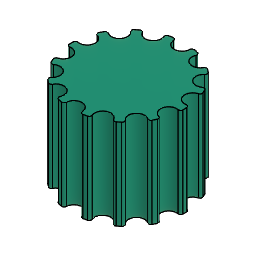
14T Pulley template v3 (Autodesk Fusion 360 design; units mm, degrees)
Autodesk Fusion 360 part; units mm, degrees
sketch "Sketch1" plane through (0, 0, 0) normal (0, 0, 1) x (1, 0, 0)
  circle A0 centre (0, 0) radius 6.305 construction
  circle A1 centre (0, 0) radius 5.105 construction
  line L0 (0, 0) -> (0, 5.105) construction
  circle A2 centre (0, 5.995) radius 0.89 construction
  circle A3 centre (1.139, 5.9469) radius 0.25 construction
  line L1 (0, 0) -> (2.7356, 5.6806) construction
  line L2 (0, 0) -> (6.305, 0) construction
  circle A4 centre (2.6011, 5.4013) radius 0.89 construction
  circle A5 centre (1.5541, 5.8522) radius 0.25 construction
  arc A6 (0.9079, 5.9375) -> (0.8892, 5.9575) centre (0, 5.105) ccw construction
  arc A7 (0, 5.105) -> (0.8892, 5.9575) centre (0, 5.995) ccw
  arc A8 (1.186, 6.1924) -> (0.8892, 5.9575) centre (1.139, 5.9469) ccw
  arc A9 (1.7837, 5.7533) -> (1.6182, 6.0938) centre (1.5541, 5.8522) ccw
  arc A10 (1.7837, 5.7533) -> (2.215, 4.5994) centre (2.6011, 5.4013) ccw
  line L3 (1.186, 6.1924) -> (1.6182, 6.0938)
  arc A11 (-0.8892, 5.9575) -> (0, 5.105) centre (0, 5.995) ccw
  arc A12 (-0.8892, 5.9575) -> (-1.186, 6.1924) centre (-1.139, 5.9469) ccw
  line L4 (-1.6182, 6.0938) -> (-1.186, 6.1924)
  arc A13 (-1.6182, 6.0938) -> (-1.7837, 5.7533) centre (-1.5541, 5.8522) ccw
  arc A14 (-2.215, 4.5994) -> (-1.7837, 5.7533) centre (-2.6011, 5.4013) ccw
  arc A15 (-3.386, 4.9817) -> (-2.215, 4.5994) centre (-2.6011, 5.4013) ccw
  arc A16 (-3.386, 4.9817) -> (-3.7554, 5.0646) centre (-3.6065, 4.8638) ccw
  line L5 (-4.102, 4.7882) -> (-3.7554, 5.0646)
  arc A17 (-4.102, 4.7882) -> (-4.1033, 4.4096) centre (-3.9393, 4.5983) ccw
  arc A18 (-3.9912, 3.1829) -> (-4.1033, 4.4096) centre (-4.6871, 3.7378) ccw
  arc A19 (-5.2121, 3.0192) -> (-3.9912, 3.1829) centre (-4.6871, 3.7378) ccw
  arc A20 (-5.2121, 3.0192) -> (-5.5809, 2.9337) centre (-5.3596, 2.8173) ccw
  line L6 (-5.7733, 2.5342) -> (-5.5809, 2.9337)
  arc A21 (-5.7733, 2.5342) -> (-5.6102, 2.1926) centre (-5.5444, 2.4337) ccw
  arc A22 (-4.977, 1.136) -> (-5.6102, 2.1926) centre (-5.8447, 1.334) ccw
  arc A23 (-6.006, 0.4587) -> (-4.977, 1.136) centre (-5.8447, 1.334) ccw
  arc A24 (-6.006, 0.4587) -> (-6.3011, 0.2217) centre (-6.0513, 0.2129) ccw
  line L7 (-6.3011, -0.2217) -> (-6.3011, 0.2217)
  arc A25 (-6.3011, -0.2217) -> (-6.006, -0.4587) centre (-6.0513, -0.2129) ccw
  arc A26 (-4.977, -1.136) -> (-6.006, -0.4587) centre (-5.8447, -1.334) ccw
  arc A27 (-5.6102, -2.1926) -> (-4.977, -1.136) centre (-5.8447, -1.334) ccw
  arc A28 (-5.6102, -2.1926) -> (-5.7733, -2.5342) centre (-5.5444, -2.4337) ccw
  line L8 (-5.5809, -2.9337) -> (-5.7733, -2.5342)
  arc A29 (-5.5809, -2.9337) -> (-5.2121, -3.0192) centre (-5.3596, -2.8173) ccw
  arc A30 (-3.9912, -3.1829) -> (-5.2121, -3.0192) centre (-4.6871, -3.7378) ccw
  arc A31 (-4.1033, -4.4096) -> (-3.9912, -3.1829) centre (-4.6871, -3.7378) ccw
  arc A32 (-4.1033, -4.4096) -> (-4.102, -4.7882) centre (-3.9393, -4.5983) ccw
  line L9 (-3.7554, -5.0646) -> (-4.102, -4.7882)
  arc A33 (-3.7554, -5.0646) -> (-3.386, -4.9817) centre (-3.6065, -4.8638) ccw
  arc A34 (-2.215, -4.5994) -> (-3.386, -4.9817) centre (-2.6011, -5.4013) ccw
  arc A35 (-1.7837, -5.7533) -> (-2.215, -4.5994) centre (-2.6011, -5.4013) ccw
  arc A36 (-1.7837, -5.7533) -> (-1.6182, -6.0938) centre (-1.5541, -5.8522) ccw
  line L10 (-1.186, -6.1924) -> (-1.6182, -6.0938)
  arc A37 (-1.186, -6.1924) -> (-0.8892, -5.9575) centre (-1.139, -5.9469) ccw
  arc A38 (0, -5.105) -> (-0.8892, -5.9575) centre (0, -5.995) ccw
  arc A39 (0.8892, -5.9575) -> (0, -5.105) centre (0, -5.995) ccw
  arc A40 (0.8892, -5.9575) -> (1.186, -6.1924) centre (1.139, -5.9469) ccw
  line L11 (1.6182, -6.0938) -> (1.186, -6.1924)
  arc A41 (1.6182, -6.0938) -> (1.7837, -5.7533) centre (1.5541, -5.8522) ccw
  arc A42 (2.215, -4.5994) -> (1.7837, -5.7533) centre (2.6011, -5.4013) ccw
  arc A43 (3.386, -4.9817) -> (2.215, -4.5994) centre (2.6011, -5.4013) ccw
  arc A44 (3.386, -4.9817) -> (3.7554, -5.0646) centre (3.6065, -4.8638) ccw
  line L12 (4.102, -4.7882) -> (3.7554, -5.0646)
  arc A45 (4.102, -4.7882) -> (4.1033, -4.4096) centre (3.9393, -4.5983) ccw
  arc A46 (3.9912, -3.1829) -> (4.1033, -4.4096) centre (4.6871, -3.7378) ccw
  arc A47 (5.2121, -3.0192) -> (3.9912, -3.1829) centre (4.6871, -3.7378) ccw
  arc A48 (5.2121, -3.0192) -> (5.5809, -2.9337) centre (5.3596, -2.8173) ccw
  line L13 (5.7733, -2.5342) -> (5.5809, -2.9337)
  arc A49 (5.7733, -2.5342) -> (5.6102, -2.1926) centre (5.5444, -2.4337) ccw
  arc A50 (4.977, -1.136) -> (5.6102, -2.1926) centre (5.8447, -1.334) ccw
  arc A51 (6.006, -0.4587) -> (4.977, -1.136) centre (5.8447, -1.334) ccw
  arc A52 (6.006, -0.4587) -> (6.3011, -0.2217) centre (6.0513, -0.2129) ccw
  line L14 (6.3011, 0.2217) -> (6.3011, -0.2217)
  arc A53 (6.3011, 0.2217) -> (6.006, 0.4587) centre (6.0513, 0.2129) ccw
  arc A54 (4.977, 1.136) -> (6.006, 0.4587) centre (5.8447, 1.334) ccw
  arc A55 (5.6102, 2.1926) -> (4.977, 1.136) centre (5.8447, 1.334) ccw
  arc A56 (5.6102, 2.1926) -> (5.7733, 2.5342) centre (5.5444, 2.4337) ccw
  line L15 (5.5809, 2.9337) -> (5.7733, 2.5342)
  arc A57 (5.5809, 2.9337) -> (5.2121, 3.0192) centre (5.3596, 2.8173) ccw
  arc A58 (3.9912, 3.1829) -> (5.2121, 3.0192) centre (4.6871, 3.7378) ccw
  arc A59 (4.1033, 4.4096) -> (3.9912, 3.1829) centre (4.6871, 3.7378) ccw
  arc A60 (4.1033, 4.4096) -> (4.102, 4.7882) centre (3.9393, 4.5983) ccw
  line L16 (3.7554, 5.0646) -> (4.102, 4.7882)
  arc A61 (3.7554, 5.0646) -> (3.386, 4.9817) centre (3.6065, 4.8638) ccw
  arc A62 (2.215, 4.5994) -> (3.386, 4.9817) centre (2.6011, 5.4013) ccw
  dimension "d1" = 12.61
  dimension "d2" = 10.21
  dimension "d3" = 1.78
  dimension "d4" = 0.5
  dimension "d6" = 25.714
  dimension "d7" = 1.78
  dimension "d8" = 0.5
  dimension "d10" = 360
  constraint coincident A0.centre A1.centre
  constraint concentric A0 A1
  constraint coincident A1 L0.end
  constraint vertical L0
  constraint coincident L0.end A2
  constraint tangent A0 A3
  constraint tangent A2 A3
  constraint tangent A1 A2
  constraint horizontal L2
  constraint coincident A0 L1.end
  constraint tangent A1 A4
  constraint coincident L1 A4.centre
  constraint tangent A4 A5
  constraint tangent A0 A5
  constraint coincident A2 A6.end
  constraint coincident A3 A6.end
  constraint coincident L0.end A6.centre
  constraint coincident A3.centre A8.centre
  constraint coincident A0 A9.end
  constraint coincident A5 A9.end
  constraint coincident A4 A9.start
  constraint coincident A5 A9.start
  constraint coincident A1 A10.end
  constraint coincident A4 A10.end
  constraint coincident L1 A10.end
  measures "d1" diameter of A0
  measures "d2" diameter of A1
  measures "d3" diameter of A2
  measures "d4" diameter of A3
  measures "d6" angle of L0 L1
  measures "d7" diameter of A4
  measures "d8" diameter of A5
extrude "Extrude1" add sketch "Sketch1" along normal blind 10
equation "d2 = d1 - ( ( 2 * 1.2 ) * 1 mm )"
equation "d7 = d3"
